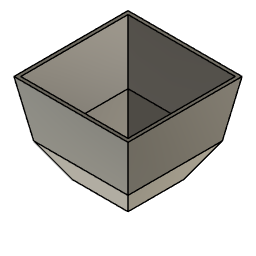
10408김준호_사각통 (Autodesk Fusion 360 design; units mm, degrees)
Autodesk Fusion 360 part; units mm, degrees
sketch "스케치1" plane through (0, 0, 0) normal (0, 0, 1) x (1, 0, 0)
  line L0 (-25, 25) -> (25, 25)
  line L1 (25, 25) -> (25, -25)
  line L2 (25, -25) -> (-25, -25)
  line L3 (-25, -25) -> (-25, 25)
  constraint horizontal L0
  constraint vertical L1
  constraint horizontal L2
  constraint vertical L3
extrude "돌출1" add sketch "스케치1" along normal blind 30 draft 30
extrude "돌출2" add 1 faces at (-14.1068, -14.1068, 30) along direction (0, 0, 1) blind 50 draft 10
shell "쉘1" thickness 3 removed faces 1 at (-17.0456, 17.0456, 80)
